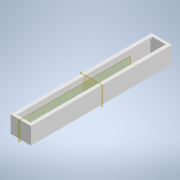
# Autodesk Inventor part: balancingFrame
Saved by Autodesk Inventor 2020 (Build 240168000, 168)
## iProperties
Created: 2022-12-14
Part Number: balancingFrame
Material: Generic
Document SubType Name: Modeling
Designer: Manish
Density: 1 g/cm^3
Appearance: Default
Author: Manish
Autodesk Inventor part; units mm, degrees
ref_plane "YZ Plane" through (0, 0, 0) normal (1, 0, 0) x (0, 1, 0)
ref_plane "XZ Plane" through (0, 0, 0) normal (0, 1, 0) x (-1, 0, 0)
ref_plane "XY Plane" through (0, 0, 0) normal (0, 0, 1) x (1, 0, 0)
sketch "Sketch1" plane through (0, 0, 0) normal (0, 0, 1) x (1, 0, 0)
  line L0 (0, 0) -> (0, -50)
  line L1 (0, -50) -> (60, -50)
  line L2 (60, -50) -> (60, 0)
  line L3 (60, 0) -> (50, 0)
  line L4 (50, 0) -> (50, -5)
  line L5 (50, -5) -> (55, -5)
  line L6 (55, -5) -> (55, -45)
  line L7 (55, -45) -> (5, -45)
  line L8 (5, -45) -> (5, -5)
  line L9 (5, -5) -> (10, -5)
  line L10 (10, -5) -> (10, 0)
  line L11 (10, 0) -> (0, 0)
  dimension "d0" = 50
  dimension "d1" = 60
  dimension "d2" = 10
  dimension "d3" = 5
  dimension "d4" = 5
  dimension "d5" = 40
  dimension "d6" = 50
  dimension "d7" = 40
  dimension "d8" = 5
  dimension "d9" = 5
  constraints: 24 end point, 8 perpendicular, 3 point on line, 1 vertical
  measures "d0" distance of L0.start L0.end
  measures "d1" distance of L0.end L1.end
  measures "d2" distance of L2.end L3.end
  measures "d3" distance of L3.end L4.end
  measures "d4" distance of L4.end L5.end
  measures "d5" distance of L5.end L6.end
  measures "d6" distance of L6.end L7.end
  measures "d7" distance of L7.end L8.end
  measures "d8" distance of L8.end L9.end
  measures "d9" distance of L9.end L10.end
extrude "Extrusion1" add sketch "Sketch1" against normal blind 400
ref_plane "Work Plane1" through (0, 0, -200) normal (0, 0, 1) x (1, 0, 0)
ref_plane "Work Plane2" through (30, -50, 0) normal (-1, 0, 0) x (0, 0, 1)
sketch "Sketch2" plane through (0, -50, 0) normal (-1, 0, 0) x (0, 0, 1)
  line L0 (0, 0) -> (-400, 0) projected
  line L1 (-400, 0) -> (-408, 0)
  line L2 (-408, 0) -> (-408, 50)
  line L3 (-408, 50) -> (-400, 50)
  line L4 (-400, 50) -> (-400, 0)
  line L5 (0, 45) -> (0, 50) projected
  line L6 (0, 50) -> (8, 50)
  line L7 (8, 50) -> (8, 0)
  line L8 (8, 0) -> (0, 0)
  line L9 (0, 0) -> (0, 50)
  dimension "d12" = 8
  dimension "d13" = 50
  dimension "d14" = 8
  constraints: 16 end point, 4 parallel, 2 horizontal, 2 perpendicular
  measures "d12" distance of L2.end L3.end
  measures "d13" distance of L1.end L2.end
  measures "d14" distance of L7.end L8.end
extrude "Extrusion2" add sketch "Sketch2" against normal blind 60
body "Solid1"
